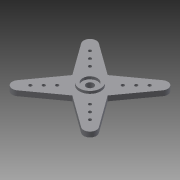
# Autodesk Inventor part: Star for servo
Saved by Autodesk Inventor 2015 (Build 190159000, 159)
## iProperties
Created: 2018-12-25
Part Number: Star for servo
Material: Типовые
Document SubType Name: Modeling
Designer: kostya
Density: 1 g/cm^3
Appearance: По умолчанию
Author: kostya
Autodesk Inventor part; units mm, degrees
ref_plane "YZ Plane" through (0, 0, 0) normal (1, 0, 0) x (0, 1, 0)
ref_plane "XZ Plane" through (0, 0, 0) normal (0, 1, 0) x (-1, 0, 0)
ref_plane "XY Plane" through (0, 0, 0) normal (0, 0, 1) x (1, 0, 0)
sketch "Эскиз1" plane through (0, 0, 0) normal (0, 0, 1) x (1, 0, 0)
  line L0 (-10, -10) -> (10, 10) construction
  line L1 (10, -10) -> (-10, 10) construction
  circle A0 centre (0, 0) radius 3.35
  line L2 (1.3848, 1.8986) -> (1.9263, 1.3461)
  line L3 (1.9263, 1.3461) -> (2.259, 0.6477)
  line L4 (2.259, 0.6477) -> (2.3469, -0.1209)
  line L5 (2.3469, -0.1209) -> (2.1805, -0.8764)
  line L6 (2.1805, -0.8764) -> (1.7778, -1.5369)
  line L7 (1.7778, -1.5369) -> (1.1824, -2.0309)
  line L8 (1.1824, -2.0309) -> (0.4589, -2.3047)
  line L9 (0.4589, -2.3047) -> (-0.3143, -2.3289)
  line L10 (-0.3143, -2.3289) -> (-1.0534, -2.1007)
  line L11 (-1.0534, -2.1007) -> (-1.6784, -1.6448)
  line L12 (-1.6784, -1.6448) -> (-2.1216, -1.0107)
  line L13 (-2.1216, -1.0107) -> (-2.3348, -0.2671)
  line L14 (-2.3348, -0.2671) -> (-2.295, 0.5055)
  line L15 (-2.295, 0.5055) -> (-2.0065, 1.2233)
  line L16 (-2.0065, 1.2233) -> (-1.5006, 1.8085)
  line L17 (-1.5006, 1.8085) -> (-0.832, 2.1978)
  line L18 (-0.832, 2.1978) -> (-0.0733, 2.3489)
  line L19 (-0.0733, 2.3489) -> (0.6933, 2.2454)
  line L20 (0.6933, 2.2454) -> (1.3848, 1.8986)
  line L21 (0, 0) -> (0, 5.6) construction
  line L22 (0, 0) -> (0, -5.6) construction
  line L23 (-5.6, -5.6) -> (5.6, -5.6) construction
  line L24 (5.6, -5.6) -> (5.6, 5.6) construction
  line L25 (5.6, 5.6) -> (-5.6, 5.6) construction
  line L26 (-5.6, 5.6) -> (-5.6, -5.6) construction
  line L27 (-5.6, -5.6) -> (5.6, 5.6) construction
  line L28 (5.6, -5.6) -> (-5.6, 5.6) construction
  line L29 (-13.3, -13.3) -> (13.3, -13.3) construction
  line L30 (13.3, -13.3) -> (13.3, 13.3) construction
  line L31 (13.3, 13.3) -> (-13.3, 13.3) construction
  line L32 (-13.3, 13.3) -> (-13.3, -13.3) construction
  line L33 (-13.3, -13.3) -> (13.3, 13.3) construction
  line L34 (13.3, -13.3) -> (-13.3, 13.3) construction
  circle A1 centre (0, 0) radius 1.15
  line L35 (13.3, 13.3) -> (9.3, 13.3) construction
  line L36 (13.3, 9.3) -> (13.3, 13.3) construction
  arc A2 (12.9209, 10.1284) -> (10.1284, 12.9209) centre (11.3, 11.3) ccw
  line L37 (0, 5.6) -> (10.1284, 12.9209)
  line L38 (5.6, 0) -> (12.9209, 10.1284)
  arc A3 (-10.1284, 12.9209) -> (-12.9209, 10.1284) centre (-11.3, 11.3) ccw
  line L39 (-5.6, 0) -> (-12.9209, 10.1284)
  line L40 (0, 5.6) -> (-10.1284, 12.9209)
  arc A4 (-12.9209, -10.1284) -> (-10.1284, -12.9209) centre (-11.3, -11.3) ccw
  line L41 (0, -5.6) -> (-10.1284, -12.9209)
  line L42 (-5.6, 0) -> (-12.9209, -10.1284)
  arc A5 (10.1284, -12.9209) -> (12.9209, -10.1284) centre (11.3, -11.3) ccw
  line L43 (5.6, 0) -> (12.9209, -10.1284)
  line L44 (0, -5.6) -> (10.1284, -12.9209)
  line L45 (-12.9209, 10.1284) -> (-5.6, 0)
  line L46 (-5.6, 0) -> (-12.9209, -10.1284)
  line L47 (-10.1284, -12.9209) -> (0, -5.6)
  line L48 (0, -5.6) -> (10.1284, -12.9209)
  line L49 (12.9209, -10.1284) -> (5.6, 0)
  line L50 (12.9209, 10.1284) -> (5.6, 0)
  line L51 (0, 5.6) -> (10.1284, 12.9209)
  arc A6 (12.9209, 10.1284) -> (10.1284, 12.9209) centre (11.3, 11.3) ccw
  arc A7 (-10.1284, 12.9209) -> (-12.9209, 10.1284) centre (-11.3, 11.3) ccw
  arc A8 (-12.9209, -10.1284) -> (-10.1284, -12.9209) centre (-11.3, -11.3) ccw
  arc A9 (10.1284, -12.9209) -> (12.9209, -10.1284) centre (11.3, -11.3) ccw
  line L52 (2.3688, 2.3688) -> (5.1972, 5.1972) construction
  circle A10 centre (5.1972, 5.1972) radius 0.5
  circle A11 centre (7.3186, 7.3186) radius 0.5
  circle A12 centre (9.4399, 9.4399) radius 0.5
  circle A13 centre (-5.1972, 5.1972) radius 0.5
  circle A14 centre (-7.3186, 7.3186) radius 0.5
  circle A15 centre (-9.4399, 9.4399) radius 0.5
  circle A16 centre (-5.1972, -5.1972) radius 0.5
  circle A17 centre (-7.3186, -7.3186) radius 0.5
  circle A18 centre (-9.4399, -9.4399) radius 0.5
  circle A19 centre (5.1972, -5.1972) radius 0.5
  circle A20 centre (7.3186, -7.3186) radius 0.5
  circle A21 centre (9.4399, -9.4399) radius 0.5
  circle A22 centre (0, 0) radius 2.3179
  dimension "d2" = 6.7
  dimension "d4" = 5.6
  dimension "d5" = 5.6
  dimension "d6" = 26.6
  dimension "d7" = 26.6
  dimension "d8" = 2.3
  dimension "d13" = 360
  dimension "d15" = 4
  dimension "d16" = 1
  dimension "d19" = 3
  dimension "d26" = 360
  constraints: 106 end point, 22 centre point, 16 point on circle, 10 coincident, 9 equal length, 9 midpoint, 7 tangent, 4 point on line, 3 concentric, 3 horizontal, 3 perpendicular, 2 vertical, 107 other
  measures "d4" distance of L21.start L21.end
  measures "d5" distance of L21.start L22.end
  measures "d6" distance of L31.end L30.end
  measures "d7" distance of L30.end L29.end
  measures "d8" diameter of A1
  measures "d15" distance of L52.start L52.end
  measures "d16" diameter of A10
  measures "d19" distance of A10.centre A11.centre
extrude "Выдавливание1" add sketch "Эскиз1" along normal mid plane 1.6 contours A22 | L38 L43 A5 L44 L41 A4 L42 L39 A3 L40 L37 A2
extrude "Выдавливание2" add sketch "Эскиз1" along normal blind 1.6 and the other way blind 2.6 contours A0
